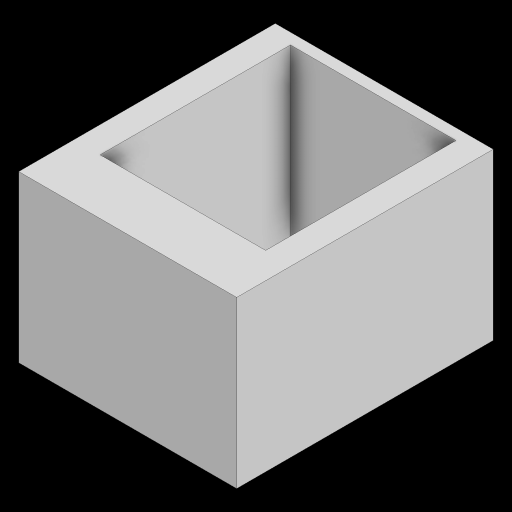
# Autodesk Inventor part: rack_supp
Saved by Autodesk Inventor 2023 (Build 270158000, 158)
## iProperties
Created: 2024-07-11
Part Number: rack_supp
Material: 일반
Document SubType Name: Modeling
Designer: OMS55
Density: 1 g/cm^3
Appearance: 기본값
Author: OMS55
Autodesk Inventor part; units mm, degrees
ref_plane "YZ Plane" through (0, 0, 0) normal (1, 0, 0) x (0, 1, 0)
ref_plane "XZ Plane" through (0, 0, 0) normal (0, 1, 0) x (-1, 0, 0)
ref_plane "XY Plane" through (0, 0, 0) normal (0, 0, 1) x (1, 0, 0)
sketch "스케치1" plane through (0, 0, 0) normal (0, 1, 0) x (-1, 0, 0)
  line L0 (30, 0) -> (0, 0)
  line L1 (0, 0) -> (0, -34.5)
  line L2 (0, -34.5) -> (30, -34.5)
  line L3 (30, -34.5) -> (30, 0)
  line L4 (34.75, 10) -> (-4.75, 10)
  line L5 (-4.75, 10) -> (-4.75, -36.5)
  line L6 (-4.75, -36.5) -> (34.75, -36.5)
  line L7 (34.75, -36.5) -> (34.75, 10)
  point P0 (15, 0)
  dimension "d0" = 30
  dimension "d1" = 34.5
  dimension "d2" = 4.75
  dimension "d3" = 4.75
  dimension "d4" = 2
  dimension "d5" = 10
  constraints: 16 end point, 4 parallel, 2 horizontal, 2 perpendicular, 1 coincident, 1 midpoint
  measures "d0" distance of L0.start L0.end
  measures "d1" distance of L2.end L0.start
  measures "d2" distance between parallel lines of L3 L7
  measures "d3" distance between parallel lines of L5 L1
  measures "d4" distance between parallel lines of L2 L6
  measures "d5" distance from line of point (15, 0) L4
extrude "돌출1" add sketch "스케치1" along normal blind 30
